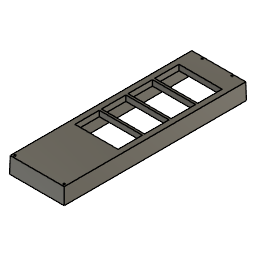
guitar (Autodesk Fusion 360 design; units mm, degrees)
part number: 2026-05-26-18-55-50-334
Autodesk Fusion 360 part; units mm, degrees
sketch "Sketch1" plane through (0, 0, 0) normal (0, 0, 1) x (1, 0, 0)
  line L0 (-23.9272, 0) -> (276.0728, 0)
  line L1 (276.0728, 0) -> (276.0728, 1000)
  line L2 (276.0728, 1000) -> (-23.9272, 1000)
  line L3 (-23.9272, 1000) -> (-23.9272, 0)
  line L4 (9.5728, 896.1324) -> (242.5728, 896.1324)
  line L5 (242.5728, 896.1324) -> (242.5728, 766.1324)
  line L6 (242.5728, 766.1324) -> (9.5728, 766.1324)
  line L7 (9.5728, 766.1324) -> (9.5728, 896.1324)
  line L8 (9.5728, 750.4224) -> (242.5728, 750.4224)
  line L9 (242.5728, 750.4224) -> (242.5728, 620.4224)
  line L10 (242.5728, 620.4224) -> (9.5728, 620.4224)
  line L11 (9.5728, 620.4224) -> (9.5728, 750.4224)
  line L12 (9.5728, 604.7124) -> (242.5728, 604.7124)
  line L13 (242.5728, 604.7124) -> (242.5728, 474.7124)
  line L14 (242.5728, 474.7124) -> (9.5728, 474.7124)
  line L15 (9.5728, 474.7124) -> (9.5728, 604.7124)
  line L16 (9.5728, 459.0024) -> (242.5728, 459.0024)
  line L17 (242.5728, 459.0024) -> (242.5728, 329.0024)
  line L18 (242.5728, 329.0024) -> (9.5728, 329.0024)
  line L19 (9.5728, 329.0024) -> (9.5728, 459.0024)
  dimension "d1" = 300
  dimension "d2" = 1000
  dimension "d3" = 130
  dimension "d4" = 130
  dimension "d5" = 233
  dimension "d6" = 233
  dimension "d7" = 33.5
  dimension "d8" = 33.5
  dimension "d9" = 15.71
  dimension "d10" = 15.71
  dimension "d11" = 15.71
  dimension "d12" = 15.71
  dimension "d13" = 15.71
  dimension "d14" = 15.71
  constraint horizontal L0
  constraint vertical L1
  constraint horizontal L2
  constraint vertical L3
  constraint horizontal L4
  constraint vertical L5
  constraint horizontal L6
  constraint vertical L7
  constraint horizontal L8
  constraint vertical L9
  constraint horizontal L10
  constraint vertical L11
  constraint horizontal L12
  constraint vertical L13
  constraint horizontal L14
  constraint vertical L15
  constraint equal L10 L12
  constraint equal L9 L13
  constraint collinear L9 L13
  constraint collinear L5 L9
  constraint horizontal L16
  constraint vertical L17
  constraint horizontal L18
  constraint vertical L19
  constraint equal L13 L17
  constraint equal L14 L16
  constraint collinear L13 L17
  measures "d1" distance of L0.start L0.end
  measures "d2" distance of L0.end L1.end
  measures "d3" distance of L4.end L5.end
  measures "d4" distance of L8.end L9.end
  measures "d5" distance of L8.start L8.end
  measures "d6" distance of L4.start L4.end
  measures "d7" distance of L1 L13
  measures "d8" distance of L3 L15
  measures "d9" distance of L14 L16
  measures "d10" distance of L10 L12
  measures "d11" distance of L6 L8
  measures "d12" distance of L14 L16
  measures "d13" distance of L10 L12
  measures "d14" distance of L6 L8
extrude "Extrude1" add sketch "Sketch1" along normal blind 100 draft -1
sketch "Sketch2" plane through (0, 0, 0) normal (0, 0, 1) x (1, 0, 0)
  line L0 (256.197, 980.5748) -> (3.983, 980.5748)
  line L1 (3.983, 980.5748) -> (3.983, 23.2664)
  line L2 (3.983, 23.2664) -> (256.197, 23.2664)
  line L3 (256.197, 23.2664) -> (256.197, 980.5748)
  constraint horizontal L0
  constraint vertical L1
  constraint horizontal L2
  constraint vertical L3
extrude "Extrude2" cut sketch "Sketch2" along normal blind 70
hole "Hole1" at (-9.3135, 14.624, 100) direction (0, 0, -1) diameter 10 depth 100 tip angle 118
sketch "Sketch3" plane through (0, 0, 100) normal (0, 0, 1) x (-1, 0, 0)
  circle A0 centre (9.3135, -14.624) radius 5
  line L0 (-7.8273, -764.3868) -> (-7.8273, -897.8779)
  line L1 (-7.8273, -897.8779) -> (-244.3183, -897.8779)
  line L2 (-244.3183, -897.8779) -> (-244.3183, -764.3868)
  line L3 (-244.3183, -764.3868) -> (-7.8273, -764.3868)
  line L4 (-7.8273, -618.6768) -> (-7.8273, -752.1679)
  line L5 (-7.8273, -752.1679) -> (-244.3183, -752.1679)
  line L6 (-244.3183, -752.1679) -> (-244.3183, -618.6768)
  line L7 (-244.3183, -618.6768) -> (-7.8273, -618.6768)
  line L8 (-7.8273, -472.9668) -> (-7.8273, -606.4579)
  line L9 (-7.8273, -606.4579) -> (-244.3183, -606.4579)
  line L10 (-244.3183, -606.4579) -> (-244.3183, -472.9668)
  line L11 (-244.3183, -472.9668) -> (-7.8273, -472.9668)
  line L12 (-7.8273, -327.2568) -> (-7.8273, -460.7479)
  line L13 (-7.8273, -460.7479) -> (-244.3183, -460.7479)
  line L14 (-244.3183, -460.7479) -> (-244.3183, -327.2568)
  line L15 (-244.3183, -327.2568) -> (-7.8273, -327.2568)
  line L16 (-274.3273, -998.2545) -> (22.1817, -998.2545)
  line L17 (22.1817, -998.2545) -> (22.1817, -1.7455)
  line L18 (22.1817, -1.7455) -> (-274.3273, -1.7455)
  line L19 (-274.3273, -1.7455) -> (-274.3273, -998.2545)
  circle A1 centre (-261.4591, -14.624) radius 5
  point P0 (-126.0728, -1.7455)
  dimension "d22" = 12.8682
  dimension "d23" = 12.8785
  constraint coincident L18 P0
  constraint equal A0 A1
  measures "d22" distance of A0.centre L17
  measures "d23" distance of A0.centre L18
hole "Hole2" at (261.4591, 14.624, 100) direction (0, 0, -1) diameter 10 depth 119 tip angle 118
hole "Hole3" at (207.9885, 988.9182, 100) direction (0, 0, -1) diameter 10 depth 120 tip angle 118
sketch "Sketch4" plane through (0, 0, 100) normal (0, 0, 1) x (-1, 0, 0)
  circle A0 centre (-207.9885, -988.9182) radius 5
  circle A1 centre (-261.4591, -14.624) radius 5
  circle A2 centre (9.3135, -14.624) radius 5
  line L0 (-7.8273, -764.3868) -> (-7.8273, -897.8779)
  line L1 (-7.8273, -897.8779) -> (-244.3183, -897.8779)
  line L2 (-244.3183, -897.8779) -> (-244.3183, -764.3868)
  line L3 (-244.3183, -764.3868) -> (-7.8273, -764.3868)
  line L4 (-7.8273, -618.6768) -> (-7.8273, -752.1679)
  line L5 (-7.8273, -752.1679) -> (-244.3183, -752.1679)
  line L6 (-244.3183, -752.1679) -> (-244.3183, -618.6768)
  line L7 (-244.3183, -618.6768) -> (-7.8273, -618.6768)
  line L8 (-7.8273, -472.9668) -> (-7.8273, -606.4579)
  line L9 (-7.8273, -606.4579) -> (-244.3183, -606.4579)
  line L10 (-244.3183, -606.4579) -> (-244.3183, -472.9668)
  line L11 (-244.3183, -472.9668) -> (-7.8273, -472.9668)
  line L12 (-7.8273, -327.2568) -> (-7.8273, -460.7479)
  line L13 (-7.8273, -460.7479) -> (-244.3183, -460.7479)
  line L14 (-244.3183, -460.7479) -> (-244.3183, -327.2568)
  line L15 (-244.3183, -327.2568) -> (-7.8273, -327.2568)
  line L16 (-274.3273, -998.2545) -> (22.1817, -998.2545)
  line L17 (22.1817, -998.2545) -> (22.1817, -1.7455)
  line L18 (22.1817, -1.7455) -> (-274.3273, -1.7455)
  line L19 (-274.3273, -1.7455) -> (-274.3273, -998.2545)
  circle A3 centre (-44.157, -988.9182) radius 5
  point P0 (-126.0728, -998.2545)
  dimension "d39" = 163.8315
  constraint coincident L16 P0
  constraint equal A0 A3
  measures "d39" distance of A0.centre A3.centre
extrude "Extrude3" cut sketch "Sketch4" against normal blind 300 contours A3
sketch "Sketch5" plane through (0, 765.899, 13.3688) normal (0, 0.999848, 0.017452) x (-1, 0, 0)
  line L0 (-243.7946, 56.6398) -> (-8.3509, 56.6398)
  line L1 (-8.3509, 56.6398) -> (-7.8273, 86.6444)
  line L2 (-7.8273, 86.6444) -> (-244.3183, 86.6444)
  line L3 (-244.3183, 86.6444) -> (-243.7946, 56.6398)
  dimension "d32" = 30.0046
  measures "d32" distance of L0 L2
sketch "Sketch6" plane through (-23.9199, 0, 0.4175) normal (-0.999848, 0, 0.017452) x (0, -1, 0)
  line L0 (-1.7455, 99.5976) -> (-998.2545, 99.5976)
  line L1 (-998.2545, 99.5976) -> (-1000, -0.4176)
  line L2 (-1000, -0.4176) -> (0, -0.4176)
  line L3 (0, -0.4176) -> (-1.7455, 99.5976)
  dimension "d33" = 100.0152
  measures "d33" distance of L0 L2
scale "Scale1" factor 0.46 about (243.7946, 473.4905, 70) bodies 1
sketch "Sketch7" plane through (0, 0, 83.8) normal (0, 0, 1) x (-1, 0, 0)
  line L0 (-257.8396, -714.8819) -> (-121.4455, -714.8819)
  line L1 (-121.4455, -714.8819) -> (-121.4455, -256.4878)
  line L2 (-121.4455, -256.4878) -> (-257.8396, -256.4878)
  line L3 (-257.8396, -256.4878) -> (-257.8396, -714.8819)
  line L4 (-135.2496, -406.223) -> (-135.2496, -467.6289)
  line L5 (-135.2496, -467.6289) -> (-244.0355, -467.6289)
  line L6 (-244.0355, -467.6289) -> (-244.0355, -406.223)
  line L7 (-244.0355, -406.223) -> (-135.2496, -406.223)
  line L8 (-135.2496, -473.2496) -> (-135.2496, -534.6555)
  line L9 (-135.2496, -534.6555) -> (-244.0355, -534.6555)
  line L10 (-244.0355, -534.6555) -> (-244.0355, -473.2496)
  line L11 (-244.0355, -473.2496) -> (-135.2496, -473.2496)
  line L12 (-135.2496, -540.2762) -> (-135.2496, -601.6821)
  line L13 (-135.2496, -601.6821) -> (-244.0355, -601.6821)
  line L14 (-244.0355, -601.6821) -> (-244.0355, -540.2762)
  line L15 (-244.0355, -540.2762) -> (-135.2496, -540.2762)
  line L16 (-135.2496, -607.3028) -> (-135.2496, -668.7087)
  line L17 (-135.2496, -668.7087) -> (-244.0355, -668.7087)
  line L18 (-244.0355, -668.7087) -> (-244.0355, -607.3028)
  line L19 (-244.0355, -607.3028) -> (-135.2496, -607.3028)
  circle A0 centre (-127.3649, -262.4119) radius 2.3
  circle A1 centre (-251.9203, -262.4119) radius 2.3
  circle A2 centre (-227.3238, -710.5872) radius 2.3
  circle A3 centre (-151.9613, -710.5872) radius 2.3
  dimension "d35" = 61.4059
  dimension "d36" = 108.7859
  measures "d35" distance of L5 L7
  measures "d36" distance of L4 L6
sketch "Sketch8" plane through (0, 716.1265, 12.5) normal (0, 0.999848, 0.017452) x (-1, 0, 0)
  line L0 (-121.4455, 71.3108) -> (-257.8396, 71.3108)
  line L1 (-257.8396, 71.3108) -> (-258.6426, 25.3038)
  line L2 (-258.6426, 25.3038) -> (-120.6426, 25.3038)
  line L3 (-120.6426, 25.3038) -> (-121.4455, 71.3108)
  line L4 (-257.8396, 71.3108) -> (-121.4455, 71.3108)
  dimension "d37" = 46.007
  measures "d37" distance of L2 L4
sketch "Sketch9" plane through (0, 0, 83.8) normal (0, 0, 1) x (-1, 0, 0)
  circle A0 centre (-151.9613, -710.5872) radius 2.3
  point P0 (-185, -715)
  point P1 (-187.4151, -715)
  point P2 (-227.3238, -710.5872)
  point P3 (-151.9613, -710.5872)
  dimension "d38" = 4.6
  dimension "d40" = 75.3625
  measures "d38" diameter of A0
  measures "d40" distance of P2 P3
sketch "Sketch10" plane through (0, 0, 83.8) normal (0, 0, 1) x (-1, 0, 0)
  line L0 (-257.8396, -256.4878) -> (-257.8396, -714.8819)
  line L1 (-121.4455, -714.8819) -> (-121.4455, -256.4878)
  line L2 (-121.4455, -256.4878) -> (-257.8396, -256.4878)
  circle A0 centre (-151.9613, -710.5872) radius 2.3
  line L3 (-257.8396, -714.8819) -> (-121.4455, -714.8819)
  point P0 (-127.3649, -262.4119)
  point P1 (-151.9613, -710.5872)
  dimension "d41" = 136.3941
  dimension "d42" = 458.3941
  dimension "d43" = 5.9194
  dimension "d44" = 5.9241
  dimension "d45" = 4.6
  dimension "d46" = 4.2947
  dimension "d47" = 30.5158
  measures "d41" distance of L0 L1
  measures "d42" distance of L1.start L1.end
  measures "d43" distance of L1 P0
  measures "d44" distance of P0 L2
  measures "d45" diameter of A0
  measures "d46" distance of P1 L3
  measures "d47" distance of L1 P1
extrude "Extrude4" cut 1 faces at (126.6208, 562.1575, 37.8) along direction (0, 0, 1) blind 5
